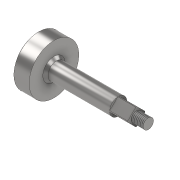
# Autodesk Inventor part: 塞杆
Saved by Autodesk Inventor 2022 (Build 260153000, 153)
## iProperties
Created: 2023-03-14
Part Number: 塞杆
Material: 不锈钢
Document SubType Name: Modeling
Designer: Lzy18
Density: 8 g/cm^3
Appearance: 半抛光
Author: Lzy18
Autodesk Inventor part; units mm, degrees
ref_plane "YZ Plane" through (0, 0, 0) normal (1, 0, 0) x (0, 1, 0)
ref_plane "XZ Plane" through (0, 0, 0) normal (0, 1, 0) x (-1, 0, 0)
ref_plane "XY Plane" through (0, 0, 0) normal (0, 0, 1) x (1, 0, 0)
sketch "草图1" plane through (0, 0, 0) normal (0, 0, 1) x (1, 0, 0)
  line L0 (0, 29) -> (0, 10)
  line L1 (0, 10) -> (75, 10)
  line L2 (0, 0) -> (110, 0)
  line L3 (110, 0) -> (110, 6)
  line L4 (110, 6) -> (75, 6)
  line L5 (75, 6) -> (75, 10)
  arc A0 (-17.749, 29) -> (-26, 15.7797) centre (14, 0) ccw
  line L6 (0, 29) -> (-17.749, 29)
  line L7 (0, 0) -> (-29, 0)
  line L8 (-26, 15.7797) -> (-26, 0)
  dimension "d0" = 110
  dimension "d1" = 10
  dimension "d2" = 6
  dimension "d4" = 86
  dimension "d5" = 29
  dimension "d8" = 35
  dimension "d14" = 26
  dimension "d15" = 14
  constraints: 18 end point, 5 perpendicular, 3 point on line, 2 horizontal, 2 point on circle, 1 centre point, 1 coincident, 1 vertical
  measures "d0" distance between parallel lines of L3 L0
  measures "d1" distance between parallel lines of L2 L1
  measures "d2" distance between parallel lines of L2 L4
  measures "d4" diameter of A0
  measures "d5" distance from line of L2 L0.start
  measures "d8" distance between parallel lines of L5 L3
  measures "d14" distance between parallel lines of L0 L8
  measures "d15" distance from line of L0 A0.centre
revolve "旋转1" add sketch "草图1" angle 360 about axis through (0, 0, 0) along (1, 0, 0)
sketch "草图2" plane through (75, 0, 0) normal (1, 0, 0) x (0, 0, -1)
  circle A0 centre (0, 0) radius 29 projected
  line L0 (0, 10.6066) -> (10.6066, 0)
  line L1 (10.6066, 0) -> (0, -10.6066)
  line L2 (0, -10.6066) -> (-10.6066, 0)
  line L3 (-10.6066, 0) -> (0, 10.6066)
  line L4 (0, 0) -> (0, 10)
  circle A1 centre (0, 0) radius 10 projected
  point P0 (0.6262, 9.9804)
  point P1 (-0.6262, 9.9804)
  point P2 (-9.9804, 0.6262)
  point P3 (-9.9804, -0.6262)
  point P4 (-0.6262, -9.9804)
  point P5 (0.6262, -9.9804)
  point P6 (9.9804, -0.6262)
  point P7 (9.9804, 0.6262)
  dimension "d9" = 7.5
  constraints: 10 end point, 1 coincident, 1 point on line, 1 vertical, 11 other
  measures "d9" distance from line of L3 point (0, 0)
extrude "拉伸1" add sketch "草图2" along normal blind 21 contours L0 A1 L1 L2 L3
thread "螺纹1" size "M12x1.75" designation "M12" class "6g" standard "GB Metric profile" full length
chamfer "倒角1" distance 3 angle 45 1 edges at (0, -10, 0)
